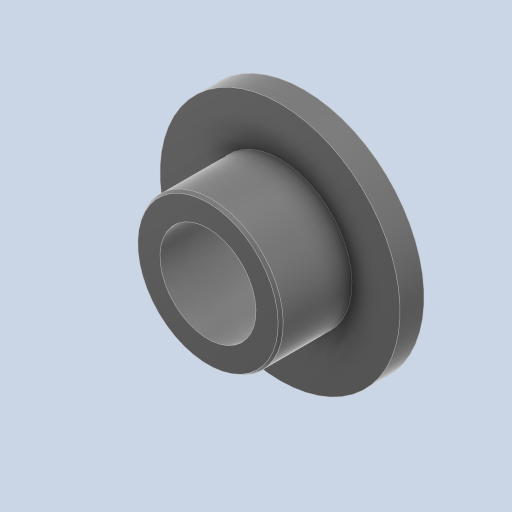
# Autodesk Inventor part: GFM-0304-03
Saved by Autodesk Inventor 2023 (Build 270158000, 158)
## iProperties
Created: 2024-11-29
Part Number: GFM-0304-03
Material: PAEK 樹脂
Document SubType Name: Modeling
Designer: kiyo
Density: 1.32 g/cm^3
Appearance: 滑らか - 黒
Author: kiyo
Autodesk Inventor part; units mm, degrees
ref_plane "YZ Plane" through (0, 0, 0) normal (1, 0, 0) x (0, 1, 0)
ref_plane "XZ Plane" through (0, 0, 0) normal (0, 1, 0) x (-1, 0, 0)
ref_plane "XY Plane" through (0, 0, 0) normal (0, 0, 1) x (1, 0, 0)
sketch "スケッチ2" plane through (0, 0, 0) normal (0, 1, 0) x (-1, 0, 0)
  line L0 (0, 1.5) -> (-0.75, 1.5)
  line L1 (-0.75, 2.25) -> (-0.75, 3.75)
  line L2 (-0.75, 3.75) -> (0, 3.75)
  line L3 (0, 3.75) -> (0, 1.5)
  line L4 (-0.75, 1.5) -> (-3, 1.5)
  line L5 (-3, 1.5) -> (-3, 2.1923)
  line L6 (0, 0) -> (-4.3872, 0)
  line L7 (-3, 2.1923) -> (-2.9, 2.25)
  line L8 (-2.9, 2.25) -> (-0.75, 2.25)
  dimension "d0" = 3.75
  dimension "d2" = 1.5
  dimension "d3" = 0.75
  dimension "d4" = 3
  dimension "d5" = 30
  dimension "d6" = 2.25
  dimension "d7" = 0.1
  dimension "d8" = 0
  constraints: 18 end point, 3 horizontal, 3 perpendicular, 2 parallel, 1 point on line
  measures "d0" distance between parallel lines of L6 L2
  measures "d2" distance between parallel lines of L6 L4
  measures "d3" distance between parallel lines of L1 L3
  measures "d4" distance between parallel lines of L5 L3
  measures "d5" angle of L7 L8
  measures "d6" distance between parallel lines of L6 L8
  measures "d7" distance from line of L7.end L5
  measures "d8" distance from line of L6.start L3
revolve "回転1" add sketch "スケッチ2" angle 360 about axis through (0, 0, 0) along (1, 0, 0)
